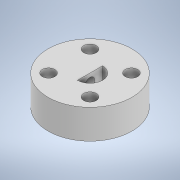
# Autodesk Inventor part: Twist_Attachment_To_Servo_Horn
Saved by Autodesk Inventor 2022 (Build 260153000, 153)
## iProperties
Created: 2022-02-26
Part Number: Twist_Attachment_To_Servo_Horn
Material: Generic
Document SubType Name: Modeling
Designer: Mlees
Density: 1 g/cm^3
Appearance: Default
Author: Mlees
Autodesk Inventor part; units mm, degrees
ref_plane "YZ Plane" through (0, 0, 0) normal (1, 0, 0) x (0, 1, 0)
ref_plane "XZ Plane" through (0, 0, 0) normal (0, 1, 0) x (-1, 0, 0)
ref_plane "XY Plane" through (0, 0, 0) normal (0, 0, 1) x (1, 0, 0)
sketch "Sketch1" plane through (0, 0, 0) normal (0, 1, 0) x (-1, 0, 0)
  circle A0 centre (0, 0) radius 10
  dimension "d0" = 20
  constraints: 1 centre point, 1 coincident
  measures "d0" diameter of A0
extrude "Extrusion1" add sketch "Sketch1" along normal blind 7
sketch "Sketch2" plane through (0, 7, 0) normal (0, 1, 0) x (1, 0, 0)
  circle A0 centre (0, 0) radius 10
  arc A1 (0, -3) -> (0, 3) centre (0, 0) ccw
  line L0 (0, -3) -> (0, 3)
  dimension "d3" = 6
  constraints: 2 centre point, 2 coincident, 2 end point, 2 point on circle, 1 vertical
  measures "d3" diameter of A1
extrude "Extrusion2" cut sketch "Sketch2" against normal blind 4 contours L0 A1
sketch "Sketch3" plane through (0, 0, 0) normal (0, -1, 0) x (1, 0, 0)
  line L0 (0, 3) -> (0, -3) projected
  circle A0 centre (0, 0) radius 3
  constraints: 1 coincident, 1 vertical alignment, 2 other
extrude "Extrusion3" cut sketch "Sketch3" against normal blind 1
ref_plane "Work Plane1" through (-10, 0, 0) normal (1, 0, 0) x (0, 0, -1)
sketch "Sketch4" plane through (-10, 0, 0) normal (1, 0, 0) x (0, 0, -1)
  line L0 (10, 7) -> (-10, 7) projected
  circle A0 centre (0, 5) radius 1.125
  point P0 (0, 0)
  dimension "d9" = 2.25
  constraints: 1 centre point
  measures "d9" diameter of A0
extrude "Extrusion4" cut sketch "Sketch4" along normal up to surface (10 mm away)
sketch "Sketch5" plane through (0, 7, 0) normal (0, 1, 0) x (1, 0, 0)
  circle A0 centre (0, 0) radius 6.985
  line L0 (0, 0) -> (6.985, 0) construction
  circle A1 centre (-4.9391, 4.9391) radius 1.5
  circle A2 centre (-4.9391, -4.9391) radius 1.5
  circle A3 centre (4.9391, -4.9391) radius 1.5
  circle A4 centre (4.9391, 4.9391) radius 1.5
  dimension "d14" = 3
  dimension "d17" = 360
  constraints: 5 centre point, 2 end point, 1 coincident, 1 horizontal, 9 other
  measures "d14" diameter of A1
extrude "Extrusion5" cut sketch "Sketch5" against normal up to surface (7 mm away) contours A4 A0 | A0 A4 | A3 A0 | A0 A3 | A1 A0 | A0 A1 | A2 A0 | A0 A2
equation "\"d19\" = d14"
body "Solid1"
